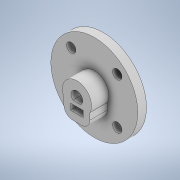
# Autodesk Inventor part: sprzeglo
Saved by Autodesk Inventor 2020 (Build 240168000, 168)
## iProperties
Created: 2020-03-28
Part Number: sprzeglo
Material: Ogólny
Document SubType Name: Modeling
Designer: niedz
Density: 1 g/cm^3
Appearance: Domyślna
Author: niedz
Autodesk Inventor part; units mm, degrees
ref_plane "YZ Plane" through (0, 0, 0) normal (1, 0, 0) x (0, 1, 0)
ref_plane "XZ Plane" through (0, 0, 0) normal (0, 1, 0) x (-1, 0, 0)
ref_plane "XY Plane" through (0, 0, 0) normal (0, 0, 1) x (1, 0, 0)
sketch "Szkic1" plane through (0, 0, 0) normal (0, 0, 1) x (1, 0, 0)
  circle A0 centre (0, 0) radius 20
  circle A1 centre (10.6, 10.6) radius 2.15
  circle A2 centre (-10.6, 10.6) radius 2.15
  circle A3 centre (-10.6, -10.6) radius 2.15
  circle A4 centre (10.6, -10.6) radius 2.15
  arc A5 (1.8342, -1.954) -> (-1.8342, -1.954) centre (0, 0) ccw
  line L0 (0, -1.954) -> (1.8342, -1.954)
  line L1 (0, -1.954) -> (-1.8342, -1.954)
  dimension "d0" = 40
  dimension "d3" = 4.3
  dimension "d6" = 360
  dimension "d8" = 5.36
  constraints: 6 centre point, 4 end point, 2 coincident, 2 point on circle, 1 horizontal, 9 other
  measures "d0" diameter of A0
  measures "d3" diameter of A1
  measures "d8" diameter of A5
extrude "Wyciągnięcie proste1" add sketch "Szkic1" along normal blind 4
sketch "Szkic2" plane through (0, 0, 4) normal (0, 0, 1) x (1, 0, 0)
  arc A0 (5.9908, -3) -> (-6.0091, -2.9632) centre (0, 0) ccw
  circle A1 centre (0, 0) radius 20 projected
  line L0 (0, -10) -> (6, -10)
  line L1 (6, -10) -> (5.9908, -3)
  line L2 (5.9908, -3) -> (-6.0091, -2.9632)
  line L3 (-6.0091, -2.9632) -> (-6.0091, -9.9632)
  line L4 (-6.0091, -9.9632) -> (0, -10)
  line L5 (-0.0091, -3.6816) -> (2.8909, -3.6816)
  line L6 (2.8909, -3.6816) -> (2.8909, -6.4816)
  line L7 (2.8909, -6.4816) -> (-2.9091, -6.4816)
  line L8 (-2.9091, -6.4816) -> (-2.9091, -3.6816)
  line L9 (-2.9091, -3.6816) -> (-0.0091, -3.6816)
  dimension "d12" = 13.4
  dimension "d19" = 6
  dimension "d20" = 7
  dimension "d21" = 12
  dimension "d24" = 7
  dimension "d26" = 2.9
  dimension "d27" = 2.8
  dimension "d28" = 5.8
  constraints: 20 end point, 4 perpendicular, 2 point on circle, 1 centre point, 1 coincident, 1 point on line, 1 vertical
  measures "d12" diameter of A0
  measures "d19" distance of L0.start L0.end
  measures "d20" distance of L0.end L1.end
  measures "d21" distance of L1.end L2.end
  measures "d24" distance of L2.end L3.end
  measures "d26" distance of L5.start L5.end
  measures "d27" distance of L5.end L6.end
  measures "d28" distance of L6.end L7.end
extrude "Wyciągnięcie proste2" add sketch "Szkic2" along normal blind 8 contours L1 L0 L4 L3 L2
sketch "Szkic3" plane through (0, 0, 4) normal (0, 0, 1) x (1, 0, 0)
  circle A0 centre (0, 0) radius 6.7
  line L0 (-6.0091, -9.9632) -> (-6.0091, -2.9632) projected
  line L1 (6, -10) -> (5.9908, -3) projected
  line L2 (-6.0091, -2.9632) -> (5.9908, -3)
  dimension "d31" = 13.4
  constraints: 2 end point, 1 centre point, 1 coincident
  measures "d31" diameter of A0
sketch "Szkic4" plane through (0, 0, 4) normal (0, 0, 1) x (1, 0, 0)
  arc A0 (1.8342, -1.954) -> (-1.8342, -1.954) centre (0, 0) ccw projected
  line L0 (-1.8342, -1.954) -> (1.8342, -1.954)
  arc A1 (1.8342, -1.954) -> (-1.8342, -1.954) centre (0, 0) ccw
  constraints: 2 end point, 2 point on circle, 1 centre point, 1 coincident, 1 concentric, 1 horizontal
sketch "Szkic5" plane through (0, 0, 4) normal (0, 0, 1) x (1, 0, 0)
  point P0 (0, 0)
extrude "Wyciągnięcie proste3" add sketch "Szkic3" along normal blind 8 contours A0 L2 picked at (-1.2468, -0.1308)
extrude "Wyciągnięcie proste4" cut sketch "Szkic4" along normal blind 8
sketch "Szkic6" plane through (0, -10, 4) normal (-0.0061262, -0.9999812, 0) x (0.9999812, -0.0061262, 0)
  circle A0 centre (0, 4) radius 1.6
  point P0 (-0.0613, -4)
  point P1 (0, 0)
  dimension "d37" = 3.2
  constraints: 1 centre point
  measures "d37" diameter of A0
extrude "Wyciągnięcie proste5" cut sketch "Szkic6" against normal blind 8
sketch "Szkic7" plane through (0.049, -2.0002, 8) normal (-0.0061262, -0.9999812, 0) x (0.9999812, -0.0061262, 0)
  point P0 (-0.0613, -8)
sketch "Szkic8" plane through (0.049, -2.0002, 8) normal (-0.0061262, -0.9999812, 0) x (0.9999812, -0.0061262, 0)
  circle A0 centre (0, 0) radius 1.6
  point P0 (-0.0613, -8)
  dimension "d40" = 3.2
  constraints: 1 centre point
  measures "d40" diameter of A0
extrude "Wyciągnięcie proste6" cut sketch "Szkic8" against normal blind 2
fillet "Zaokrąglenie1" radius 4 1 edges at (-6.0091, -9.9632, 8)
fillet "Zaokrąglenie2" radius 4 1 edges at (6, -10, 8)
sketch "Szkic9" plane through (0, -10, 8) normal (-0.0061262, -0.9999812, 0) x (0.9999812, -0.0061262, 0)
  point P0 (-0.0613, -8)
